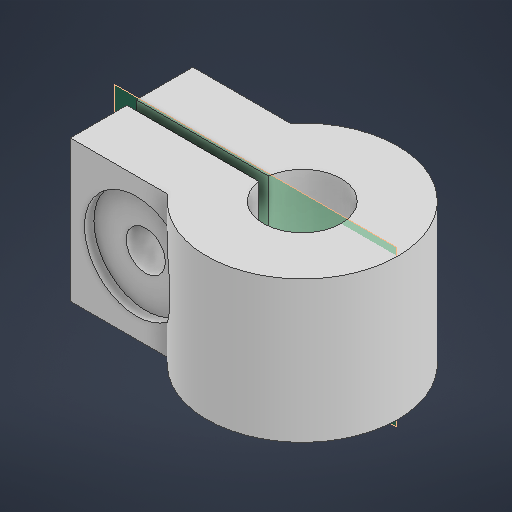
# Autodesk Inventor part: Abrazadera
Saved by Autodesk Inventor 2026.1 (Build 301233020, 233B)
## iProperties
Created: 2025-10-21
Part Number: Abrazadera
Material: Generic
Document SubType Name: Modeling
Designer: tito.luyo
Density: 1 g/cm^3
Appearance: Default
Author: tito.luyo
Autodesk Inventor part; units mm, degrees
ref_plane "YZ Plane" through (0, 0, 0) normal (1, 0, 0) x (0, 1, 0)
ref_plane "XZ Plane" through (0, 0, 0) normal (0, 1, 0) x (-1, 0, 0)
ref_plane "XY Plane" through (0, 0, 0) normal (0, 0, 1) x (1, 0, 0)
sketch "Sketch1" plane through (0, 0, 0) normal (0, 1, 0) x (-1, 0, 0)
  circle A0 centre (0, 0) radius 4.125
  circle A1 centre (0, 0) radius 10.125
  line L0 (4.0946, 0.5) -> (18.0946, 0.5)
  line L1 (18.0946, 0.5) -> (18.0946, 6.5)
  line L2 (18.0946, 6.5) -> (4.0946, 6.5)
  line L3 (4.0946, 6.5) -> (4.0946, 0.5)
  line L4 (-15, 0) -> (15, 0) construction
  line L5 (-15, 0) -> (15, 0) construction
  line L6 (4.0946, -0.5) -> (18.0946, -0.5)
  line L7 (18.0946, -0.5) -> (18.0946, -6.5)
  line L8 (18.0946, -6.5) -> (4.0946, -6.5)
  line L9 (4.0946, -6.5) -> (4.0946, -0.5)
  point P0 (7.7631, 6.5)
  point P1 (7.7631, -6.5)
  point P2 (10.1126, -0.5)
  point P3 (4.0946, -5.2082)
  point P4 (4.0946, 5.2082)
  point P5 (10.1126, 0.5)
  dimension "eje" = 8.25
  dimension "diam_externo" = 20.25
  dimension "sep" = 0.5
  dimension "guia_central" = 30
  dimension "d4" = 0
  dimension "lengueta_espesor" = 6
  dimension "lengueta_alto" = 14
  constraints: 20 end point, 4 symmetric about line, 3 horizontal, 2 coincident, 2 parallel, 1 centre point, 1 collinear, 1 perpendicular, 3 other
  measures "diam_externo" diameter of A1
  measures "sep" distance from line of point (0, 0) L0
  measures "guia_central" distance of L4.start L4.end
  measures "d4" distance between parallel lines of L4 L5
  measures "lengueta_espesor" distance between parallel lines of L2 L0
  measures "lengueta_alto" distance between parallel lines of L1 L3
extrude "abrazadera" add sketch "Sketch1" along normal blind 15 contours L3 L2 A1 L0 | A0 L9 L8 A1 L2 L3 | L6 A1 L8 L9 | A1 L2 L1 L0 | L6 L7 L8 A1
sketch "Sketch5" plane through (-7.7631, 0, -6.5) normal (0, 0, -1) x (-1, 0, 0)
  circle A0 centre (3.3315, 7.6408) radius 2.075
  line L0 (-3.6685, 0) -> (-3.6685, 15) projected
  point P0 (-7.7631, 0)
  dimension "hueco_tornillo" = 4.15
  dimension "hueco_tornillo_distancia" = 7
  constraints: 1 centre point
  measures "hueco_tornillo" diameter of A0
  measures "hueco_tornillo_distancia" distance from line of L0 A0.centre
extrude "tornillo" cut sketch "Sketch5" against normal blind 13
sketch "Sketch6" plane through (-7.7631, 0, -6.5) normal (0, 0, -1) x (-1, 0, 0)
  circle A0 centre (3.3315, 7.6408) radius 2.075 projected
  circle A1 centre (3.3315, 7.6408) radius 5.5
  point P0 (-7.7631, 0)
  dimension "arandela" = 11
  constraints: 1 centre point, 1 coincident
  measures "arandela" diameter of A1
extrude "arandela" cut sketch "Sketch6" along normal blind 5 and the other way blind 1
ref_plane "Work Plane1" through (-7.7631, 0, 0) normal (0, 0, -1) x (-1, 0, 0)
mirror "Mirror1" about plane through (-7.7631, 0, 0) normal (0, 0, -1) of "arandela"
equation "\"diam_externo\" = eje + 2 * espesor"
equation "\"lengueta_espesor\" = espesor"
equation "\"hueco_tornillo_agujero\" = 2 * sep + 2 * lengueta_espesor"
equation "\"espesor\" = 6"
body "Solid2"
